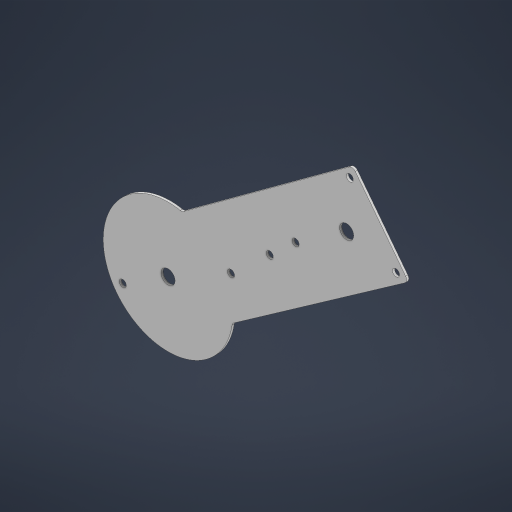
# Autodesk Inventor part: Intake poly
Saved by Autodesk Inventor 2023.4 (Build 274418000, 418)
## iProperties
Created: 2023-12-15
Part Number: Intake poly
Material: Generic
Document SubType Name: Modeling
Designer: diego
Density: 1 g/cm^3
Appearance: Default
Author: diego
Autodesk Inventor part; units mm, degrees
ref_plane "YZ Plane" through (0, 0, 0) normal (1, 0, 0) x (0, 1, 0)
ref_plane "XZ Plane" through (0, 0, 0) normal (0, 1, 0) x (-1, 0, 0)
ref_plane "XY Plane" through (0, 0, 0) normal (0, 0, 1) x (1, 0, 0)
sketch "Sketch1" plane through (0, 0, 0) normal (0, 0, 1) x (1, 0, 0)
  circle A0 centre (-409.232, 138.4433) radius 46.99
  line L0 (-362.6127, 132.5526) -> (-234.9094, 222.3444)
  line L1 (-234.9094, 222.3444) -> (-275.3173, 274.9342)
  line L2 (-275.3173, 274.9342) -> (-399.0023, 184.3063)
  circle A1 centre (-316.7088, 206.2787) radius 2.54
  circle A2 centre (-335.4324, 189.1151) radius 2.54
  circle A3 centre (-363.5177, 163.3697) radius 2.54
  circle A4 centre (-243.9143, 223.6901) radius 2.54
  circle A5 centre (-277.3954, 266.5628) radius 2.54
  circle A6 centre (-279.6641, 231.5651) radius 5.08
  circle A7 centre (-409.232, 138.4433) radius 5.08
  circle A8 centre (-442.0215, 117.854) radius 2.54
  point P0 (0, 0)
  dimension "d31" = 93.98
  dimension "d32" = 127.7033
  dimension "d33" = 153.3343
  dimension "d34" = 5.08
  dimension "d35" = 5.08
  dimension "d36" = 5.08
  dimension "d37" = 5.08
  dimension "d38" = 5.08
  dimension "d39" = 10.16
  dimension "d40" = 10.16
  dimension "d41" = 5.08
  constraints: 9 centre point, 6 end point, 2 point on circle, 1 coincident
  measures "d31" diameter of A0
  measures "d32" horizontal distance of L0.start L0.end
  measures "d33" distance of L1.end L2.end
  measures "d34" diameter of A1
  measures "d35" diameter of A2
  measures "d36" diameter of A3
  measures "d37" diameter of A4
  measures "d38" diameter of A5
  measures "d39" diameter of A6
  measures "d40" diameter of A7
  measures "d41" diameter of A8
extrude "Extrusion1" add sketch "Sketch1" along normal blind 1.5875
fillet "Fillet1" radius 3.175 4 edges at (-275.3173, 274.9342, 0.7937) (-234.9094, 222.3444, 0.7937) (-362.6127, 132.5526, 0.7937) (-399.0023, 184.3063, 0.7937)
body "Solid1"
